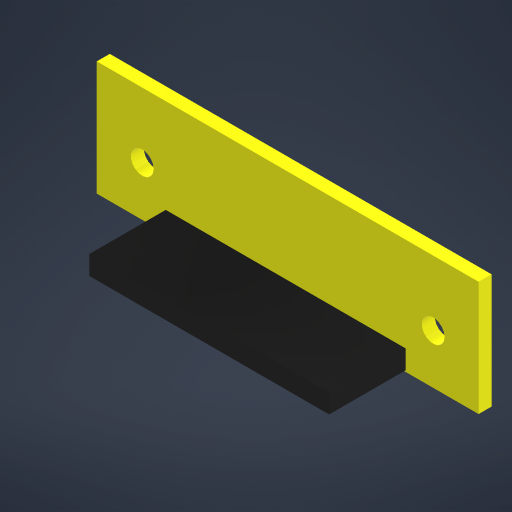
# Autodesk Inventor part: DeviceConnector
Saved by Autodesk Inventor 2024.2 (Build 282272000, 272)
## iProperties
Created: 2024-06-03
Part Number: DeviceConnector
Material: Generic
Document SubType Name: Modeling
Designer: simon
Density: 1 g/cm^3
Appearance: Default
Author: simon
Autodesk Inventor part; units mm, degrees
ref_plane "YZ Plane" through (0, 0, 0) normal (1, 0, 0) x (0, 1, 0)
ref_plane "XZ Plane" through (0, 0, 0) normal (0, 1, 0) x (-1, 0, 0)
ref_plane "XY Plane" through (0, 0, 0) normal (0, 0, 1) x (1, 0, 0)
sketch "Sketch1" plane through (0, 0, 0) normal (0, 0, 1) x (1, 0, 0)
  line L0 (0, 0) -> (50, 0)
  line L1 (50, 0) -> (50, 15)
  line L2 (50, 15) -> (0, 15)
  line L3 (0, 15) -> (0, 0)
  circle A0 centre (5.95, 6.5) radius 1.5
  circle A1 centre (44.05, 6.5) radius 1.5
  dimension "d0" = 50
  dimension "d1" = 15
  dimension "d4" = 3
  dimension "d5" = 3
  dimension "d6" = 38.1
  dimension "d7" = 5.95
  dimension "d8" = 6.5
  dimension "d9" = 6.5
  constraints: 8 end point, 2 centre point, 2 parallel, 1 horizontal, 1 perpendicular
  measures "d0" distance of L2.end L1.end
  measures "d1" distance of L1.end L0.end
  measures "d4" diameter of A0
  measures "d5" diameter of A1
  measures "d6" distance of A1.centre A0.centre
  measures "d7" distance from line of L3 A0.centre
  measures "d8" distance from line of A1.centre L0
  measures "d9" distance from line of L0 A0.centre
extrude "Extrusion1" add sketch "Sketch1" along normal blind 1.7
sketch "Sketch2" plane through (0, 0, 1.7) normal (0, 0, 1) x (1, 0, 0)
  line L0 (9.03, 2.67) -> (40.43, 2.67)
  line L1 (40.43, 2.67) -> (40.43, 0.17)
  line L2 (40.43, 0.17) -> (9.03, 0.17)
  line L3 (9.03, 0.17) -> (9.03, 2.67)
  circle A0 centre (5.95, 6.5) radius 1.5 projected
  point P0 (0, 0)
  dimension "d10" = 31.4
  dimension "d11" = 2.5
  dimension "d12" = 3.83
  dimension "d13" = 3.08
  constraints: 8 end point, 2 parallel, 1 horizontal, 1 perpendicular
  measures "d10" distance of L1.end L2.end
  measures "d11" distance of L0.end L1.end
  measures "d12" distance from line of A0.centre L0
  measures "d13" distance from line of L3 A0.centre
extrude "Extrusion2" add sketch "Sketch2" along normal blind 10 contours L0 L1 L2 L3
body "Solid1"
